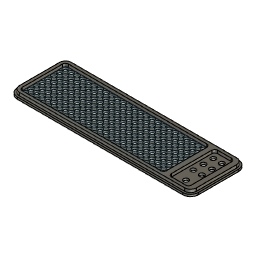
Frontal (Autodesk Fusion 360 design; units mm, degrees)
Autodesk Fusion 360 part; units mm, degrees
sketch "Boceto1" plane through (0, 0, 0) normal (0, 0, 1) x (1, 0, 0)
  circle A0 centre (2.9, 2.9) radius 2.5
  circle A1 centre (8.7, 2.9) radius 2.5
  circle A2 centre (20.3, 2.9) radius 2.5
  circle A3 centre (14.5, 2.9) radius 2.5
  circle A4 centre (43.5, 2.9) radius 2.5
  circle A5 centre (26.1, 2.9) radius 2.5
  circle A6 centre (31.9, 2.9) radius 2.5
  circle A7 centre (37.7, 2.9) radius 2.5
  circle A8 centre (55.1, 2.9) radius 2.5
  circle A9 centre (78.3, 2.9) radius 2.5
  circle A10 centre (84.1, 2.9) radius 2.5
  circle A11 centre (72.5, 2.9) radius 2.5
  circle A12 centre (89.9, 2.9) radius 2.5
  circle A13 centre (60.9, 2.9) radius 2.5
  circle A14 centre (66.7, 2.9) radius 2.5
  circle A15 centre (49.3, 2.9) radius 2.5
  circle A16 centre (118.9, 2.9) radius 2.5
  circle A17 centre (107.3, 2.9) radius 2.5
  circle A18 centre (95.7, 2.9) radius 2.5
  circle A19 centre (136.3, 2.9) radius 2.5
  circle A20 centre (113.1, 2.9) radius 2.5
  circle A21 centre (130.5, 2.9) radius 2.5
  circle A22 centre (124.7, 2.9) radius 2.5
  circle A23 centre (142.1, 2.9) radius 2.5
  circle A24 centre (101.5, 2.9) radius 2.5
  circle A25 centre (142.1, 8.7) radius 2.5
  circle A26 centre (66.7, 8.7) radius 2.5
  circle A27 centre (60.9, 8.7) radius 2.5
  circle A28 centre (2.9, 8.7) radius 2.5
  circle A29 centre (72.5, 8.7) radius 2.5
  circle A30 centre (130.5, 8.7) radius 2.5
  circle A31 centre (43.5, 8.7) radius 2.5
  circle A32 centre (20.3, 8.7) radius 2.5
  circle A33 centre (31.9, 8.7) radius 2.5
  circle A34 centre (101.5, 8.7) radius 2.5
  circle A35 centre (84.1, 8.7) radius 2.5
  circle A36 centre (113.1, 8.7) radius 2.5
  circle A37 centre (8.7, 8.7) radius 2.5
  circle A38 centre (55.1, 8.7) radius 2.5
  circle A39 centre (78.3, 8.7) radius 2.5
  circle A40 centre (124.7, 8.7) radius 2.5
  circle A41 centre (14.5, 8.7) radius 2.5
  circle A42 centre (26.1, 8.7) radius 2.5
  circle A43 centre (49.3, 8.7) radius 2.5
  circle A44 centre (89.9, 8.7) radius 2.5
  circle A45 centre (37.7, 8.7) radius 2.5
  circle A46 centre (136.3, 8.7) radius 2.5
  circle A47 centre (118.9, 8.7) radius 2.5
  circle A48 centre (107.3, 8.7) radius 2.5
  circle A49 centre (95.7, 8.7) radius 2.5
  circle A50 centre (78.3, 14.5) radius 2.5
  circle A51 centre (72.5, 14.5) radius 2.5
  circle A52 centre (26.1, 14.5) radius 2.5
  circle A53 centre (136.3, 20.3) radius 2.5
  circle A54 centre (37.7, 20.3) radius 2.5
  circle A55 centre (89.9, 20.3) radius 2.5
  circle A56 centre (49.3, 20.3) radius 2.5
  circle A57 centre (66.7, 14.5) radius 2.5
  circle A58 centre (113.1, 20.3) radius 2.5
  circle A59 centre (118.9, 20.3) radius 2.5
  circle A60 centre (124.7, 20.3) radius 2.5
  circle A61 centre (84.1, 20.3) radius 2.5
  circle A62 centre (20.3, 14.5) radius 2.5
  circle A63 centre (72.5, 20.3) radius 2.5
  circle A64 centre (142.1, 14.5) radius 2.5
  circle A65 centre (55.1, 14.5) radius 2.5
  circle A66 centre (14.5, 14.5) radius 2.5
  circle A67 centre (8.7, 20.3) radius 2.5
  circle A68 centre (101.5, 14.5) radius 2.5
  circle A69 centre (118.9, 14.5) radius 2.5
  circle A70 centre (2.9, 14.5) radius 2.5
  circle A71 centre (107.3, 14.5) radius 2.5
  circle A72 centre (8.7, 14.5) radius 2.5
  circle A73 centre (124.7, 14.5) radius 2.5
  circle A74 centre (113.1, 14.5) radius 2.5
  circle A75 centre (26.1, 20.3) radius 2.5
  circle A76 centre (49.3, 14.5) radius 2.5
  circle A77 centre (20.3, 20.3) radius 2.5
  circle A78 centre (66.7, 20.3) radius 2.5
  circle A79 centre (43.5, 14.5) radius 2.5
  circle A80 centre (43.5, 20.3) radius 2.5
  circle A81 centre (130.5, 20.3) radius 2.5
  circle A82 centre (78.3, 20.3) radius 2.5
  circle A83 centre (31.9, 14.5) radius 2.5
  circle A84 centre (89.9, 14.5) radius 2.5
  circle A85 centre (95.7, 20.3) radius 2.5
  circle A86 centre (55.1, 20.3) radius 2.5
  circle A87 centre (37.7, 14.5) radius 2.5
  circle A88 centre (31.9, 20.3) radius 2.5
  circle A89 centre (107.3, 20.3) radius 2.5
  circle A90 centre (101.5, 20.3) radius 2.5
  circle A91 centre (60.9, 20.3) radius 2.5
  circle A92 centre (130.5, 14.5) radius 2.5
  circle A93 centre (84.1, 14.5) radius 2.5
  circle A94 centre (14.5, 20.3) radius 2.5
  circle A95 centre (60.9, 14.5) radius 2.5
  circle A96 centre (2.9, 20.3) radius 2.5
  circle A97 centre (136.3, 14.5) radius 2.5
  circle A98 centre (142.1, 20.3) radius 2.5
  circle A99 centre (95.7, 14.5) radius 2.5
  circle A100 centre (55.1, 26.1) radius 2.5
  circle A101 centre (31.9, 31.9) radius 2.5
  circle A102 centre (95.7, 26.1) radius 2.5
  circle A103 centre (136.3, 26.1) radius 2.5
  circle A104 centre (43.5, 26.1) radius 2.5
  circle A105 centre (60.9, 26.1) radius 2.5
  circle A106 centre (8.7, 26.1) radius 2.5
  circle A107 centre (113.1, 31.9) radius 2.5
  circle A108 centre (49.3, 31.9) radius 2.5
  circle A109 centre (84.1, 26.1) radius 2.5
  circle A110 centre (49.3, 26.1) radius 2.5
  circle A111 centre (89.9, 26.1) radius 2.5
  circle A112 centre (130.5, 31.9) radius 2.5
  circle A113 centre (101.5, 31.9) radius 2.5
  circle A114 centre (31.9, 26.1) radius 2.5
  circle A115 centre (142.1, 31.9) radius 2.5
  circle A116 centre (8.7, 31.9) radius 2.5
  circle A117 centre (72.5, 26.1) radius 2.5
  circle A118 centre (78.3, 31.9) radius 2.5
  circle A119 centre (124.7, 31.9) radius 2.5
  circle A120 centre (118.9, 26.1) radius 2.5
  circle A121 centre (78.3, 26.1) radius 2.5
  circle A122 centre (66.7, 31.9) radius 2.5
  circle A123 centre (113.1, 26.1) radius 2.5
  circle A124 centre (142.1, 26.1) radius 2.5
  circle A125 centre (26.1, 31.9) radius 2.5
  circle A126 centre (60.9, 31.9) radius 2.5
  circle A127 centre (89.9, 31.9) radius 2.5
  circle A128 centre (26.1, 26.1) radius 2.5
  circle A129 centre (37.7, 26.1) radius 2.5
  circle A130 centre (72.5, 31.9) radius 2.5
  circle A131 centre (20.3, 26.1) radius 2.5
  circle A132 centre (14.5, 26.1) radius 2.5
  circle A133 centre (84.1, 31.9) radius 2.5
  circle A134 centre (136.3, 31.9) radius 2.5
  circle A135 centre (14.5, 31.9) radius 2.5
  circle A136 centre (124.7, 26.1) radius 2.5
  circle A137 centre (66.7, 26.1) radius 2.5
  circle A138 centre (101.5, 26.1) radius 2.5
  circle A139 centre (118.9, 31.9) radius 2.5
  circle A140 centre (43.5, 31.9) radius 2.5
  circle A141 centre (107.3, 31.9) radius 2.5
  circle A142 centre (55.1, 31.9) radius 2.5
  circle A143 centre (107.3, 26.1) radius 2.5
  circle A144 centre (20.3, 31.9) radius 2.5
  circle A145 centre (2.9, 31.9) radius 2.5
  circle A146 centre (2.9, 26.1) radius 2.5
  circle A147 centre (130.5, 26.1) radius 2.5
  circle A148 centre (95.7, 31.9) radius 2.5
  circle A149 centre (37.7, 31.9) radius 2.5
  circle A150 centre (84.1, 43.5) radius 2.5
  circle A151 centre (84.1, 37.7) radius 2.5
  circle A152 centre (72.5, 43.5) radius 2.5
  circle A153 centre (78.3, 37.7) radius 2.5
  circle A154 centre (89.9, 37.7) radius 2.5
  circle A155 centre (72.5, 37.7) radius 2.5
  circle A156 centre (78.3, 43.5) radius 2.5
  circle A157 centre (89.9, 43.5) radius 2.5
  circle A158 centre (95.7, 37.7) radius 2.5
  circle A159 centre (107.3, 37.7) radius 2.5
  circle A160 centre (107.3, 43.5) radius 2.5
  circle A161 centre (14.5, 37.7) radius 2.5
  circle A162 centre (43.5, 37.7) radius 2.5
  circle A163 centre (31.9, 43.5) radius 2.5
  circle A164 centre (66.7, 37.7) radius 2.5
  circle A165 centre (124.7, 43.5) radius 2.5
  circle A166 centre (101.5, 43.5) radius 2.5
  circle A167 centre (95.7, 43.5) radius 2.5
  circle A168 centre (8.7, 43.5) radius 2.5
  circle A169 centre (26.1, 37.7) radius 2.5
  circle A170 centre (113.1, 37.7) radius 2.5
  circle A171 centre (20.3, 43.5) radius 2.5
  circle A172 centre (113.1, 43.5) radius 2.5
  circle A173 centre (49.3, 37.7) radius 2.5
  circle A174 centre (37.7, 37.7) radius 2.5
  circle A175 centre (49.3, 43.5) radius 2.5
  circle A176 centre (2.9, 43.5) radius 2.5
  circle A177 centre (130.5, 43.5) radius 2.5
  circle A178 centre (118.9, 43.5) radius 2.5
  circle A179 centre (55.1, 43.5) radius 2.5
  circle A180 centre (66.7, 43.5) radius 2.5
  circle A181 centre (136.3, 43.5) radius 2.5
  circle A182 centre (60.9, 43.5) radius 2.5
  circle A183 centre (136.3, 37.7) radius 2.5
  circle A184 centre (142.1, 43.5) radius 2.5
  circle A185 centre (43.5, 43.5) radius 2.5
  circle A186 centre (101.5, 37.7) radius 2.5
  circle A187 centre (2.9, 37.7) radius 2.5
  circle A188 centre (20.3, 37.7) radius 2.5
  circle A189 centre (130.5, 37.7) radius 2.5
  circle A190 centre (14.5, 43.5) radius 2.5
  circle A191 centre (37.7, 43.5) radius 2.5
  circle A192 centre (118.9, 37.7) radius 2.5
  circle A193 centre (55.1, 37.7) radius 2.5
  circle A194 centre (31.9, 37.7) radius 2.5
  circle A195 centre (124.7, 37.7) radius 2.5
  circle A196 centre (60.9, 37.7) radius 2.5
  circle A197 centre (142.1, 37.7) radius 2.5
  circle A198 centre (26.1, 43.5) radius 2.5
  circle A199 centre (8.7, 37.7) radius 2.5
  line L0 (2.9, 0) -> (142.1, 0)
  line L1 (145, 2.9) -> (145, 43.5)
  line L2 (0, 43.5) -> (0, 2.9)
  line L3 (-2.9, 43.5) -> (-2.9, 2.9)
  line L4 (2.9, -2.9) -> (169.2, -2.9)
  line L5 (142.1, 46.4) -> (2.9, 46.4)
  line L6 (175, 2.9) -> (175, 43.5)
  line L7 (169.2, 49.3) -> (2.9, 49.3)
  arc A200 (2.9, 49.3) -> (-2.9, 43.5) centre (2.9, 43.5) ccw
  arc A201 (-2.9, 2.9) -> (2.9, -2.9) centre (2.9, 2.9) ccw
  arc A202 (169.2, -2.9) -> (175, 2.9) centre (169.2, 2.9) ccw
  arc A203 (175, 43.5) -> (169.2, 49.3) centre (169.2, 43.5) ccw
  arc A204 (2.9, 46.4) -> (0, 43.5) centre (2.9, 43.5) ccw
  arc A205 (0, 2.9) -> (2.9, 0) centre (2.9, 2.9) ccw
  arc A206 (142.1, 0) -> (145, 2.9) centre (142.1, 2.9) ccw
  arc A207 (145, 43.5) -> (142.1, 46.4) centre (142.1, 43.5) ccw
  line L8 (170, 2.4388) -> (170, 43.0388)
  line L9 (166.6388, 46.4) -> (152.9, 46.4)
  arc A208 (170, 43.0388) -> (166.6388, 46.4) centre (166.6388, 43.0388) ccw
  arc A209 (167.5612, 0) -> (170, 2.4388) centre (167.5612, 2.4388) ccw
  line L10 (152.9, 0) -> (167.5612, 0)
  line L11 (150, 43.5) -> (150, 2.9)
  arc A210 (152.9, 46.4) -> (150, 43.5) centre (152.9, 43.5) ccw
  arc A211 (150, 2.9) -> (152.9, 0) centre (152.9, 2.9) ccw
  circle A212 centre (155, 20) radius 2.5
  circle A213 centre (155, 30) radius 2.5
  circle A214 centre (155, 40) radius 2.5
  circle A215 centre (160, 7.5) radius 2.5
  circle A216 centre (155, 20) radius 2.5
  circle A217 centre (155, 30) radius 2.5
  circle A218 centre (155, 40) radius 2.5
  circle A219 centre (163.5, 20) radius 2.5
  circle A220 centre (163.5, 30) radius 2.5
  circle A221 centre (163.5, 40) radius 2.5
  circle A222 centre (101.5, 120.3) radius 2.5
  circle A223 centre (89.9, 126.1) radius 2.5
  line L12 (2.9, 97.1) -> (169.2, 97.1)
  circle A224 centre (89.9, 114.5) radius 2.5
  line L13 (142.1, 146.4) -> (2.9, 146.4)
  circle A225 centre (95.7, 120.3) radius 2.5
  circle A226 centre (95.7, 143.5) radius 2.5
  circle A227 centre (89.9, 143.5) radius 2.5
  circle A228 centre (101.5, 114.5) radius 2.5
  circle A229 centre (55.1, 137.7) radius 2.5
  circle A230 centre (107.3, 102.9) radius 2.5
  circle A231 centre (43.5, 126.1) radius 2.5
  circle A232 centre (55.1, 131.9) radius 2.5
  circle A233 centre (101.5, 108.7) radius 2.5
  circle A234 centre (89.9, 137.7) radius 2.5
  circle A235 centre (101.5, 102.9) radius 2.5
  circle A236 centre (107.3, 108.7) radius 2.5
  circle A237 centre (124.7, 114.5) radius 2.5
  circle A238 centre (2.9, 126.1) radius 2.5
  circle A239 centre (124.7, 131.9) radius 2.5
  circle A240 centre (60.9, 102.9) radius 2.5
  circle A241 centre (84.1, 126.1) radius 2.5
  circle A242 centre (78.3, 114.5) radius 2.5
  circle A243 centre (155, 130) radius 2.5
  circle A244 centre (136.3, 143.5) radius 2.5
  circle A245 centre (118.9, 114.5) radius 2.5
  circle A246 centre (14.5, 131.9) radius 2.5
  circle A247 centre (113.1, 143.5) radius 2.5
  circle A248 centre (155, 140) radius 2.5
  circle A249 centre (163.5, 130) radius 2.5
  circle A250 centre (130.5, 120.3) radius 2.5
  circle A251 centre (142.1, 143.5) radius 2.5
  circle A252 centre (136.3, 114.5) radius 2.5
  circle A253 centre (26.1, 126.1) radius 2.5
  circle A254 centre (130.5, 126.1) radius 2.5
  arc A255 (-2.9, 102.9) -> (2.9, 97.1) centre (2.9, 102.9) ccw
  circle A256 centre (101.5, 126.1) radius 2.5
  circle A257 centre (142.1, 102.9) radius 2.5
  circle A258 centre (142.1, 131.9) radius 2.5
  circle A259 centre (160, 107.5) radius 2.5
  circle A260 centre (78.3, 102.9) radius 2.5
  circle A261 centre (49.3, 120.3) radius 2.5
  circle A262 centre (118.9, 137.7) radius 2.5
  circle A263 centre (20.3, 137.7) radius 2.5
  circle A264 centre (142.1, 120.3) radius 2.5
  circle A265 centre (26.1, 131.9) radius 2.5
  circle A266 centre (118.9, 126.1) radius 2.5
  circle A267 centre (142.1, 137.7) radius 2.5
  line L14 (170, 102.4388) -> (170, 143.0388)
  circle A268 centre (124.7, 143.5) radius 2.5
  arc A269 (2.9, 149.3) -> (-2.9, 143.5) centre (2.9, 143.5) ccw
  circle A270 centre (118.9, 120.3) radius 2.5
  circle A271 centre (130.5, 108.7) radius 2.5
  circle A272 centre (8.7, 108.7) radius 2.5
  circle A273 centre (118.9, 131.9) radius 2.5
  circle A274 centre (8.7, 126.1) radius 2.5
  circle A275 centre (66.7, 114.5) radius 2.5
  circle A276 centre (84.1, 108.7) radius 2.5
  circle A277 centre (8.7, 131.9) radius 2.5
  circle A278 centre (113.1, 131.9) radius 2.5
  arc A279 (142.1, 100) -> (145, 102.9) centre (142.1, 102.9) ccw
  circle A280 centre (31.9, 120.3) radius 2.5
  circle A281 centre (142.1, 108.7) radius 2.5
  line L15 (-2.9, 143.5) -> (-2.9, 102.9)
  circle A282 centre (2.9, 137.7) radius 2.5
  circle A283 centre (136.3, 102.9) radius 2.5
  circle A284 centre (8.7, 120.3) radius 2.5
  circle A285 centre (20.3, 108.7) radius 2.5
  circle A286 centre (31.9, 131.9) radius 2.5
  circle A287 centre (136.3, 120.3) radius 2.5
  circle A288 centre (130.5, 131.9) radius 2.5
  circle A289 centre (155, 120) radius 2.5
  circle A290 centre (14.5, 137.7) radius 2.5
  circle A291 centre (130.5, 114.5) radius 2.5
  circle A292 centre (26.1, 102.9) radius 2.5
  circle A293 centre (14.5, 108.7) radius 2.5
  circle A294 centre (14.5, 102.9) radius 2.5
  circle A295 centre (20.3, 102.9) radius 2.5
  circle A296 centre (2.9, 108.7) radius 2.5
  arc A297 (167.5612, 100) -> (170, 102.4388) centre (167.5612, 102.4388) ccw
  circle A298 centre (124.7, 102.9) radius 2.5
  arc A299 (150, 102.9) -> (152.9, 100) centre (152.9, 102.9) ccw
  circle A300 centre (26.1, 120.3) radius 2.5
  circle A301 centre (31.9, 108.7) radius 2.5
  circle A302 centre (26.1, 114.5) radius 2.5
  circle A303 centre (113.1, 108.7) radius 2.5
  arc A304 (169.2, 97.1) -> (175, 102.9) centre (169.2, 102.9) ccw
  line L16 (152.9, 100) -> (167.5612, 100)
  circle A305 centre (118.9, 108.7) radius 2.5
  circle A306 centre (20.3, 120.3) radius 2.5
  circle A307 centre (8.7, 102.9) radius 2.5
  circle A308 centre (163.5, 120) radius 2.5
  circle A309 centre (8.7, 114.5) radius 2.5
  arc A310 (175, 143.5) -> (169.2, 149.3) centre (169.2, 143.5) ccw
  circle A311 centre (118.9, 102.9) radius 2.5
  circle A312 centre (113.1, 120.3) radius 2.5
  circle A313 centre (124.7, 120.3) radius 2.5
  arc A314 (0, 102.9) -> (2.9, 100) centre (2.9, 102.9) ccw
  circle A315 centre (20.3, 114.5) radius 2.5
  circle A316 centre (155, 120) radius 2.5
  circle A317 centre (136.3, 137.7) radius 2.5
  circle A318 centre (124.7, 126.1) radius 2.5
  circle A319 centre (14.5, 120.3) radius 2.5
  circle A320 centre (163.5, 140) radius 2.5
  circle A321 centre (136.3, 131.9) radius 2.5
  circle A322 centre (14.5, 114.5) radius 2.5
  circle A323 centre (130.5, 102.9) radius 2.5
  circle A324 centre (136.3, 108.7) radius 2.5
  circle A325 centre (124.7, 137.7) radius 2.5
  circle A326 centre (124.7, 108.7) radius 2.5
  circle A327 centre (142.1, 114.5) radius 2.5
  circle A328 centre (26.1, 108.7) radius 2.5
  circle A329 centre (118.9, 143.5) radius 2.5
  circle A330 centre (155, 140) radius 2.5
  circle A331 centre (31.9, 114.5) radius 2.5
  circle A332 centre (2.9, 114.5) radius 2.5
  circle A333 centre (2.9, 120.3) radius 2.5
  circle A334 centre (113.1, 114.5) radius 2.5
  arc A335 (170, 143.0388) -> (166.6388, 146.4) centre (166.6388, 143.0388) ccw
  circle A336 centre (95.7, 137.7) radius 2.5
  circle A337 centre (66.7, 108.7) radius 2.5
  circle A338 centre (130.5, 143.5) radius 2.5
  circle A339 centre (43.5, 143.5) radius 2.5
  circle A340 centre (78.3, 120.3) radius 2.5
  circle A341 centre (37.7, 114.5) radius 2.5
  line L17 (175, 102.9) -> (175, 143.5)
  circle A342 centre (37.7, 137.7) radius 2.5
  circle A343 centre (66.7, 143.5) radius 2.5
  circle A344 centre (60.9, 126.1) radius 2.5
  circle A345 centre (55.1, 126.1) radius 2.5
  circle A346 centre (20.3, 131.9) radius 2.5
  circle A347 centre (84.1, 143.5) radius 2.5
  circle A348 centre (101.5, 143.5) radius 2.5
  circle A349 centre (95.7, 114.5) radius 2.5
  circle A350 centre (2.9, 143.5) radius 2.5
  circle A351 centre (49.3, 102.9) radius 2.5
  arc A352 (145, 143.5) -> (142.1, 146.4) centre (142.1, 143.5) ccw
  circle A353 centre (14.5, 143.5) radius 2.5
  circle A354 centre (84.1, 102.9) radius 2.5
  circle A355 centre (60.9, 143.5) radius 2.5
  circle A356 centre (107.3, 143.5) radius 2.5
  circle A357 centre (60.9, 120.3) radius 2.5
  circle A358 centre (49.3, 131.9) radius 2.5
  circle A359 centre (55.1, 108.7) radius 2.5
  circle A360 centre (2.9, 131.9) radius 2.5
  circle A361 centre (142.1, 126.1) radius 2.5
  circle A362 centre (43.5, 108.7) radius 2.5
  circle A363 centre (60.9, 137.7) radius 2.5
  circle A364 centre (107.3, 137.7) radius 2.5
  circle A365 centre (8.7, 137.7) radius 2.5
  circle A366 centre (49.3, 143.5) radius 2.5
  circle A367 centre (60.9, 131.9) radius 2.5
  circle A368 centre (72.5, 137.7) radius 2.5
  circle A369 centre (72.5, 114.5) radius 2.5
  circle A370 centre (55.1, 102.9) radius 2.5
  circle A371 centre (89.9, 131.9) radius 2.5
  circle A372 centre (72.5, 131.9) radius 2.5
  circle A373 centre (72.5, 120.3) radius 2.5
  circle A374 centre (66.7, 120.3) radius 2.5
  circle A375 centre (95.7, 131.9) radius 2.5
  line L18 (166.6388, 146.4) -> (152.9, 146.4)
  circle A376 centre (66.7, 102.9) radius 2.5
  circle A377 centre (26.1, 143.5) radius 2.5
  line L19 (0, 143.5) -> (0, 102.9)
  circle A378 centre (84.1, 120.3) radius 2.5
  circle A379 centre (43.5, 114.5) radius 2.5
  arc A380 (152.9, 146.4) -> (150, 143.5) centre (152.9, 143.5) ccw
  circle A381 centre (20.3, 126.1) radius 2.5
  line L20 (150, 143.5) -> (150, 102.9)
  line L21 (145, 102.9) -> (145, 143.5)
  circle A382 centre (37.7, 102.9) radius 2.5
  circle A383 centre (37.7, 120.3) radius 2.5
  circle A384 centre (26.1, 137.7) radius 2.5
  circle A385 centre (31.9, 126.1) radius 2.5
  circle A386 centre (66.7, 137.7) radius 2.5
  circle A387 centre (37.7, 143.5) radius 2.5
  circle A388 centre (31.9, 143.5) radius 2.5
  circle A389 centre (101.5, 137.7) radius 2.5
  circle A390 centre (55.1, 143.5) radius 2.5
  circle A391 centre (113.1, 137.7) radius 2.5
  circle A392 centre (84.1, 114.5) radius 2.5
  circle A393 centre (43.5, 120.3) radius 2.5
  circle A394 centre (72.5, 102.9) radius 2.5
  circle A395 centre (155, 130) radius 2.5
  circle A396 centre (78.3, 126.1) radius 2.5
  circle A397 centre (37.7, 108.7) radius 2.5
  circle A398 centre (66.7, 131.9) radius 2.5
  circle A399 centre (49.3, 108.7) radius 2.5
  circle A400 centre (43.5, 131.9) radius 2.5
  circle A401 centre (72.5, 126.1) radius 2.5
  circle A402 centre (101.5, 131.9) radius 2.5
  circle A403 centre (49.3, 126.1) radius 2.5
  arc A404 (2.9, 146.4) -> (0, 143.5) centre (2.9, 143.5) ccw
  circle A405 centre (113.1, 126.1) radius 2.5
  circle A406 centre (78.3, 131.9) radius 2.5
  circle A407 centre (78.3, 143.5) radius 2.5
  circle A408 centre (43.5, 102.9) radius 2.5
  circle A409 centre (72.5, 143.5) radius 2.5
  circle A410 centre (84.1, 131.9) radius 2.5
  circle A411 centre (43.5, 137.7) radius 2.5
  circle A412 centre (78.3, 137.7) radius 2.5
  circle A413 centre (31.9, 137.7) radius 2.5
  circle A414 centre (49.3, 137.7) radius 2.5
  circle A415 centre (20.3, 143.5) radius 2.5
  circle A416 centre (55.1, 114.5) radius 2.5
  circle A417 centre (89.9, 108.7) radius 2.5
  circle A418 centre (107.3, 120.3) radius 2.5
  circle A419 centre (72.5, 108.7) radius 2.5
  circle A420 centre (49.3, 114.5) radius 2.5
  circle A421 centre (130.5, 137.7) radius 2.5
  circle A422 centre (8.7, 143.5) radius 2.5
  circle A423 centre (136.3, 126.1) radius 2.5
  circle A424 centre (60.9, 108.7) radius 2.5
  circle A425 centre (78.3, 108.7) radius 2.5
  circle A426 centre (95.7, 126.1) radius 2.5
  circle A427 centre (107.3, 131.9) radius 2.5
  circle A428 centre (60.9, 114.5) radius 2.5
  circle A429 centre (37.7, 126.1) radius 2.5
  circle A430 centre (66.7, 126.1) radius 2.5
  circle A431 centre (14.5, 126.1) radius 2.5
  circle A432 centre (107.3, 126.1) radius 2.5
  circle A433 centre (37.7, 131.9) radius 2.5
  circle A434 centre (55.1, 120.3) radius 2.5
  circle A435 centre (84.1, 137.7) radius 2.5
  circle A436 centre (2.9, 102.9) radius 2.5
  circle A437 centre (31.9, 102.9) radius 2.5
  circle A438 centre (113.1, 102.9) radius 2.5
  circle A439 centre (89.9, 120.3) radius 2.5
  line L22 (169.2, 149.3) -> (2.9, 149.3)
  line L23 (2.9, 100) -> (142.1, 100)
  circle A440 centre (95.7, 108.7) radius 2.5
  circle A441 centre (89.9, 102.9) radius 2.5
  circle A442 centre (95.7, 102.9) radius 2.5
  circle A443 centre (107.3, 114.5) radius 2.5
  point P0 (0, 100)
  constraint horizontal L0
  constraint vertical L1
  constraint vertical L2
  constraint vertical L3
  constraint horizontal L4
  constraint horizontal L5
  constraint vertical L6
  constraint horizontal L7
  constraint tangent L3 A200
  constraint tangent L7 A200
  constraint tangent L4 A201
  constraint tangent L3 A201
  constraint tangent L4 A202
  constraint tangent L6 A202
  constraint tangent L7 A203
  constraint tangent L6 A203
  constraint tangent L2 A204
  constraint tangent L5 A204
  constraint tangent L2 A205
  constraint tangent L0 A205
  constraint tangent L0 A206
  constraint tangent L1 A206
  constraint tangent L5 A207
  constraint tangent L1 A207
  constraint horizontal L10
  constraint vertical L8
  constraint horizontal L9
  constraint tangent A209 L10
  constraint tangent L8 A209
  constraint tangent L9 A208
  constraint tangent L8 A208
  constraint vertical L11
  constraint tangent L11 A210
  constraint tangent L11 A211
  constraint coincident L0 L10.start
  constraint horizontal L23
  constraint vertical L21
  constraint vertical L19
  constraint vertical L15
  constraint horizontal L12
  constraint horizontal L13
  constraint vertical L17
  constraint horizontal L22
  constraint tangent A269 L15
  constraint tangent A269 L22
  constraint tangent L12 A255
  constraint tangent A255 L15
  constraint tangent L12 A304
  constraint tangent A304 L17
  constraint tangent A310 L22
  constraint tangent A310 L17
  constraint tangent L19 A404
  constraint tangent L13 A404
  constraint tangent A314 L19
  constraint tangent A314 L23
  constraint tangent A279 L23
  constraint tangent A279 L21
  constraint tangent L13 A352
  constraint tangent A352 L21
  constraint horizontal L16
  constraint vertical L14
  constraint horizontal L18
  constraint tangent A297 L16
  constraint tangent L14 A297
  constraint tangent A335 L18
  constraint tangent L14 A335
  constraint vertical L20
  constraint tangent A380 L20
  constraint tangent A299 L20
  constraint coincident A299.end L23
extrude "Extruir1" add sketch "Boceto1" along normal blind 2 contours L3 L4 L6 L7 A200 A201 A202 A203 | L13 A279 A314 A352 L19 L21 A404 L23 | L14 A297 A299 L16 A335 L18 A380 L20 makes body 1 at (173.3333, 29.8129, 0) makes body 2 at (133.0442, 111.9999, 0) makes body 3 at (153.787, 109.6573, 0)
extrude "Extruir2" add 1 faces at (173.3333, 29.8129, 2) along direction (0, 0, 1) blind 3 on bodies 1 bodies 1
move_body "Desplazar1" bodies 2 3 to x (1, 0, 0) y (0, 1, 0) z (0, 0, 1) at (0, -100, 0)
combine "Combinar1" operation add target body 2 tool bodies 1 3
sketch "Boceto2" plane through (0, 0, 2) normal (0, 0, 1) x (-1, 0, 0)
  circle A0 centre (-101.5, -8.7) radius 2.5
  circle A1 centre (-2.9, -14.5) radius 2.5
  circle A2 centre (-37.7, -8.7) radius 2.5
  circle A3 centre (-142.1, -26.1) radius 2.5
  circle A4 centre (-136.3, -26.1) radius 2.5
  circle A5 centre (-78.3, -20.3) radius 2.5
  circle A6 centre (-60.9, -2.9) radius 2.5
  circle A7 centre (-43.5, -43.5) radius 2.5
  circle A8 centre (-130.5, -43.5) radius 2.5
  circle A9 centre (-43.5, -2.9) radius 2.5
  circle A10 centre (-43.5, -31.9) radius 2.5
  circle A11 centre (-107.3, -31.9) radius 2.5
  circle A12 centre (-66.7, -8.7) radius 2.5
  circle A13 centre (-95.7, -37.7) radius 2.5
  circle A14 centre (-118.9, -37.7) radius 2.5
  circle A15 centre (-49.3, -20.3) radius 2.5
  circle A16 centre (-20.3, -26.1) radius 2.5
  circle A17 centre (-66.7, -37.7) radius 2.5
  circle A18 centre (-124.7, -14.5) radius 2.5
  circle A19 centre (-113.1, -14.5) radius 2.5
  circle A20 centre (-2.9, -20.3) radius 2.5
  circle A21 centre (-31.9, -14.5) radius 2.5
  circle A22 centre (-31.9, -43.5) radius 2.5
  circle A23 centre (-72.5, -43.5) radius 2.5
  circle A24 centre (-118.9, -26.1) radius 2.5
  circle A25 centre (-95.7, -26.1) radius 2.5
  circle A26 centre (-118.9, -43.5) radius 2.5
  circle A27 centre (-26.1, -8.7) radius 2.5
  circle A28 centre (-55.1, -31.9) radius 2.5
  circle A29 centre (-107.3, -20.3) radius 2.5
  circle A30 centre (-142.1, -14.5) radius 2.5
  circle A31 centre (-118.9, -14.5) radius 2.5
  circle A32 centre (-124.7, -8.7) radius 2.5
  circle A33 centre (-72.5, -20.3) radius 2.5
  circle A34 centre (-124.7, -37.7) radius 2.5
  circle A35 centre (-84.1, -31.9) radius 2.5
  circle A36 centre (-136.3, -8.7) radius 2.5
  circle A37 centre (-130.5, -2.9) radius 2.5
  circle A38 centre (-101.5, -20.3) radius 2.5
  circle A39 centre (-14.5, -14.5) radius 2.5
  circle A40 centre (-60.9, -8.7) radius 2.5
  circle A41 centre (-43.5, -8.7) radius 2.5
  circle A42 centre (-136.3, -31.9) radius 2.5
  circle A43 centre (-72.5, -8.7) radius 2.5
  circle A44 centre (-107.3, -8.7) radius 2.5
  circle A45 centre (-124.7, -43.5) radius 2.5
  circle A46 centre (-72.5, -31.9) radius 2.5
  circle A47 centre (-14.5, -20.3) radius 2.5
  circle A48 centre (-66.7, -20.3) radius 2.5
  circle A49 centre (-124.7, -26.1) radius 2.5
  circle A50 centre (-72.5, -2.9) radius 2.5
  circle A51 centre (-26.1, -31.9) radius 2.5
  circle A52 centre (-136.3, -37.7) radius 2.5
  circle A53 centre (-37.7, -20.3) radius 2.5
  circle A54 centre (-101.5, -37.7) radius 2.5
  circle A55 centre (-20.3, -14.5) radius 2.5
  circle A56 centre (-60.9, -20.3) radius 2.5
  circle A57 centre (-142.1, -2.9) radius 2.5
  circle A58 centre (-124.7, -20.3) radius 2.5
  circle A59 centre (-89.9, -26.1) radius 2.5
  circle A60 centre (-8.7, -43.5) radius 2.5
  circle A61 centre (-60.9, -37.7) radius 2.5
  circle A62 centre (-113.1, -20.3) radius 2.5
  circle A63 centre (-130.5, -37.7) radius 2.5
  circle A64 centre (-89.9, -31.9) radius 2.5
  circle A65 centre (-118.9, -2.9) radius 2.5
  circle A66 centre (-84.1, -26.1) radius 2.5
  circle A67 centre (-118.9, -31.9) radius 2.5
  circle A68 centre (-95.7, -31.9) radius 2.5
  circle A69 centre (-8.7, -14.5) radius 2.5
  circle A70 centre (-113.1, -43.5) radius 2.5
  circle A71 centre (-43.5, -20.3) radius 2.5
  circle A72 centre (-113.1, -37.7) radius 2.5
  circle A73 centre (-8.7, -2.9) radius 2.5
  circle A74 centre (-101.5, -2.9) radius 2.5
  circle A75 centre (-20.3, -20.3) radius 2.5
  circle A76 centre (-130.5, -8.7) radius 2.5
  circle A77 centre (-118.9, -8.7) radius 2.5
  circle A78 centre (-8.7, -37.7) radius 2.5
  circle A79 centre (-101.5, -26.1) radius 2.5
  circle A80 centre (-49.3, -31.9) radius 2.5
  circle A81 centre (-113.1, -8.7) radius 2.5
  circle A82 centre (-55.1, -14.5) radius 2.5
  circle A83 centre (-95.7, -20.3) radius 2.5
  circle A84 centre (-26.1, -14.5) radius 2.5
  circle A85 centre (-31.9, -8.7) radius 2.5
  circle A86 centre (-55.1, -2.9) radius 2.5
  circle A87 centre (-55.1, -37.7) radius 2.5
  circle A88 centre (-84.1, -20.3) radius 2.5
  circle A89 centre (-26.1, -20.3) radius 2.5
  circle A90 centre (-43.5, -26.1) radius 2.5
  circle A91 centre (-124.7, -2.9) radius 2.5
  circle A92 centre (-2.9, -8.7) radius 2.5
  circle A93 centre (-136.3, -43.5) radius 2.5
  circle A94 centre (-31.9, -37.7) radius 2.5
  circle A95 centre (-43.5, -37.7) radius 2.5
  circle A96 centre (-20.3, -2.9) radius 2.5
  circle A97 centre (-2.9, -26.1) radius 2.5
  circle A98 centre (-43.5, -14.5) radius 2.5
  circle A99 centre (-95.7, -43.5) radius 2.5
  circle A100 centre (-14.5, -2.9) radius 2.5
  circle A101 centre (-55.1, -8.7) radius 2.5
  circle A102 centre (-14.5, -8.7) radius 2.5
  circle A103 centre (-26.1, -37.7) radius 2.5
  circle A104 centre (-26.1, -2.9) radius 2.5
  circle A105 centre (-130.5, -14.5) radius 2.5
  circle A106 centre (-66.7, -14.5) radius 2.5
  circle A107 centre (-49.3, -14.5) radius 2.5
  circle A108 centre (-14.5, -26.1) radius 2.5
  circle A109 centre (-14.5, -37.7) radius 2.5
  circle A110 centre (-8.7, -8.7) radius 2.5
  circle A111 centre (-89.9, -37.7) radius 2.5
  circle A112 centre (-72.5, -14.5) radius 2.5
  circle A113 centre (-130.5, -31.9) radius 2.5
  circle A114 centre (-14.5, -31.9) radius 2.5
  circle A115 centre (-136.3, -20.3) radius 2.5
  circle A116 centre (-49.3, -8.7) radius 2.5
  circle A117 centre (-101.5, -14.5) radius 2.5
  circle A118 centre (-14.5, -43.5) radius 2.5
  circle A119 centre (-84.1, -14.5) radius 2.5
  circle A120 centre (-101.5, -31.9) radius 2.5
  circle A121 centre (-84.1, -2.9) radius 2.5
  circle A122 centre (-49.3, -37.7) radius 2.5
  circle A123 centre (-37.7, -26.1) radius 2.5
  circle A124 centre (-95.7, -2.9) radius 2.5
  circle A125 centre (-95.7, -8.7) radius 2.5
  circle A126 centre (-89.9, -20.3) radius 2.5
  circle A127 centre (-113.1, -2.9) radius 2.5
  circle A128 centre (-107.3, -26.1) radius 2.5
  circle A129 centre (-2.9, -2.9) radius 2.5
  circle A130 centre (-89.9, -2.9) radius 2.5
  circle A131 centre (-84.1, -37.7) radius 2.5
  circle A132 centre (-37.7, -31.9) radius 2.5
  circle A133 centre (-55.1, -20.3) radius 2.5
  circle A134 centre (-31.9, -2.9) radius 2.5
  circle A135 centre (-107.3, -14.5) radius 2.5
  circle A136 centre (-101.5, -43.5) radius 2.5
  circle A137 centre (-20.3, -37.7) radius 2.5
  circle A138 centre (-107.3, -43.5) radius 2.5
  circle A139 centre (-26.1, -26.1) radius 2.5
  circle A140 centre (-8.7, -31.9) radius 2.5
  circle A141 centre (-107.3, -2.9) radius 2.5
  circle A142 centre (-84.1, -8.7) radius 2.5
  circle A143 centre (-142.1, -8.7) radius 2.5
  circle A144 centre (-55.1, -43.5) radius 2.5
  circle A145 centre (-113.1, -26.1) radius 2.5
  circle A146 centre (-78.3, -37.7) radius 2.5
  circle A147 centre (-66.7, -31.9) radius 2.5
  circle A148 centre (-136.3, -2.9) radius 2.5
  circle A149 centre (-72.5, -37.7) radius 2.5
  circle A150 centre (-84.1, -43.5) radius 2.5
  circle A151 centre (-49.3, -2.9) radius 2.5
  circle A152 centre (-113.1, -31.9) radius 2.5
  circle A153 centre (-78.3, -31.9) radius 2.5
  circle A154 centre (-78.3, -43.5) radius 2.5
  circle A155 centre (-66.7, -26.1) radius 2.5
  circle A156 centre (-49.3, -43.5) radius 2.5
  circle A157 centre (-31.9, -26.1) radius 2.5
  circle A158 centre (-2.9, -31.9) radius 2.5
  circle A159 centre (-31.9, -31.9) radius 2.5
  circle A160 centre (-37.7, -2.9) radius 2.5
  circle A161 centre (-89.9, -14.5) radius 2.5
  circle A162 centre (-95.7, -14.5) radius 2.5
  circle A163 centre (-78.3, -8.7) radius 2.5
  circle A164 centre (-66.7, -2.9) radius 2.5
  circle A165 centre (-130.5, -20.3) radius 2.5
  circle A166 centre (-37.7, -37.7) radius 2.5
  circle A167 centre (-60.9, -43.5) radius 2.5
  circle A168 centre (-78.3, -2.9) radius 2.5
  circle A169 centre (-89.9, -8.7) radius 2.5
  circle A170 centre (-20.3, -31.9) radius 2.5
  circle A171 centre (-60.9, -31.9) radius 2.5
  circle A172 centre (-31.9, -20.3) radius 2.5
  circle A173 centre (-60.9, -26.1) radius 2.5
  circle A174 centre (-49.3, -26.1) radius 2.5
  circle A175 centre (-124.7, -31.9) radius 2.5
  circle A176 centre (-107.3, -37.7) radius 2.5
  circle A177 centre (-130.5, -26.1) radius 2.5
  circle A178 centre (-37.7, -14.5) radius 2.5
  circle A179 centre (-142.1, -37.7) radius 2.5
  circle A180 centre (-78.3, -14.5) radius 2.5
  circle A181 centre (-8.7, -20.3) radius 2.5
  circle A182 centre (-142.1, -43.5) radius 2.5
  circle A183 centre (-78.3, -26.1) radius 2.5
  circle A184 centre (-136.3, -14.5) radius 2.5
  circle A185 centre (-8.7, -26.1) radius 2.5
  circle A186 centre (-26.1, -43.5) radius 2.5
  circle A187 centre (-55.1, -26.1) radius 2.5
  circle A188 centre (-60.9, -14.5) radius 2.5
  circle A189 centre (-66.7, -43.5) radius 2.5
  circle A190 centre (-142.1, -31.9) radius 2.5
  circle A191 centre (-72.5, -26.1) radius 2.5
  circle A192 centre (-37.7, -43.5) radius 2.5
  circle A193 centre (-2.9, -37.7) radius 2.5
  circle A194 centre (-20.3, -8.7) radius 2.5
  circle A195 centre (-2.9, -43.5) radius 2.5
  circle A196 centre (-20.3, -43.5) radius 2.5
  circle A197 centre (-89.9, -43.5) radius 2.5
  circle A198 centre (-142.1, -20.3) radius 2.5
  circle A199 centre (-118.9, -20.3) radius 2.5
  line L0 (-2.9, 0) -> (-142.1, 0)
  arc A200 (-142.1, 0) -> (-145, -2.9) centre (-142.1, -2.9) ccw
  line L1 (-145, -2.9) -> (-145, -43.5)
  arc A201 (-145, -43.5) -> (-142.1, -46.4) centre (-142.1, -43.5) ccw
  line L2 (-142.1, -46.4) -> (-2.9, -46.4)
  arc A202 (-2.9, -46.4) -> (0, -43.5) centre (-2.9, -43.5) ccw
  line L3 (0, -43.5) -> (0, -2.9)
  arc A203 (0, -2.9) -> (-2.9, 0) centre (-2.9, -2.9) ccw
sketch "Boceto3" plane through (0, 0, 0) normal (0, 0, 1) x (1, 0, 0)
sketch "Boceto4" plane through (0, 0, 0) normal (0, 0, 1) x (1, 0, 0)
  circle A0 centre (26.1, 14.5) radius 2.5
  circle A1 centre (8.7, 20.3) radius 2.5
  line L0 (152.9, 0) -> (167.5612, 0)
  circle A2 centre (155, 20) radius 2.5
  circle A3 centre (130.5, 20.3) radius 2.5
  circle A4 centre (2.9, 2.9) radius 2.5
  circle A5 centre (160, 7.5) radius 2.5
  circle A6 centre (130.5, 2.9) radius 2.5
  circle A7 centre (14.5, 2.9) radius 2.5
  circle A8 centre (37.7, 20.3) radius 2.5
  circle A9 centre (136.3, 20.3) radius 2.5
  arc A10 (142.1, 0) -> (145, 2.9) centre (142.1, 2.9) ccw
  arc A11 (0, 2.9) -> (2.9, 0) centre (2.9, 2.9) ccw
  circle A12 centre (8.7, 14.5) radius 2.5
  circle A13 centre (20.3, 20.3) radius 2.5
  circle A14 centre (8.7, 8.7) radius 2.5
  circle A15 centre (8.7, 2.9) radius 2.5
  circle A16 centre (78.3, 2.9) radius 2.5
  circle A17 centre (84.1, 8.7) radius 2.5
  circle A18 centre (130.5, 8.7) radius 2.5
  circle A19 centre (95.7, 20.3) radius 2.5
  circle A20 centre (37.7, 14.5) radius 2.5
  circle A21 centre (142.1, 2.9) radius 2.5
  circle A22 centre (31.9, 14.5) radius 2.5
  circle A23 centre (142.1, 8.7) radius 2.5
  circle A24 centre (95.7, 2.9) radius 2.5
  circle A25 centre (20.3, 14.5) radius 2.5
  circle A26 centre (60.9, 14.5) radius 2.5
  circle A27 centre (89.9, 2.9) radius 2.5
  circle A28 centre (2.9, 20.3) radius 2.5
  arc A29 (-2.9, 2.9) -> (2.9, -2.9) centre (2.9, 2.9) ccw
  circle A30 centre (95.7, 43.5) radius 2.5
  circle A31 centre (31.9, 31.9) radius 2.5
  circle A32 centre (124.7, 31.9) radius 2.5
  circle A33 centre (142.1, 20.3) radius 2.5
  circle A34 centre (26.1, 20.3) radius 2.5
  circle A35 centre (89.9, 14.5) radius 2.5
  circle A36 centre (124.7, 20.3) radius 2.5
  circle A37 centre (37.7, 2.9) radius 2.5
  circle A38 centre (2.9, 14.5) radius 2.5
  circle A39 centre (136.3, 2.9) radius 2.5
  circle A40 centre (107.3, 14.5) radius 2.5
  circle A41 centre (95.7, 26.1) radius 2.5
  circle A42 centre (136.3, 8.7) radius 2.5
  arc A43 (150, 2.9) -> (152.9, 0) centre (152.9, 2.9) ccw
  circle A44 centre (26.1, 31.9) radius 2.5
  circle A45 centre (14.5, 37.7) radius 2.5
  circle A46 centre (20.3, 2.9) radius 2.5
  circle A47 centre (113.1, 2.9) radius 2.5
  circle A48 centre (31.9, 2.9) radius 2.5
  circle A49 centre (26.1, 8.7) radius 2.5
  circle A50 centre (142.1, 14.5) radius 2.5
  circle A51 centre (14.5, 14.5) radius 2.5
  circle A52 centre (31.9, 20.3) radius 2.5
  circle A53 centre (113.1, 43.5) radius 2.5
  circle A54 centre (60.9, 20.3) radius 2.5
  circle A55 centre (43.5, 31.9) radius 2.5
  circle A56 centre (26.1, 2.9) radius 2.5
  arc A57 (167.5612, 0) -> (170, 2.4388) centre (167.5612, 2.4388) ccw
  circle A58 centre (55.1, 37.7) radius 2.5
  circle A59 centre (124.7, 2.9) radius 2.5
  circle A60 centre (136.3, 26.1) radius 2.5
  circle A61 centre (49.3, 14.5) radius 2.5
  circle A62 centre (136.3, 31.9) radius 2.5
  circle A63 centre (89.9, 26.1) radius 2.5
  circle A64 centre (130.5, 43.5) radius 2.5
  circle A65 centre (72.5, 20.3) radius 2.5
  circle A66 centre (78.3, 26.1) radius 2.5
  circle A67 centre (113.1, 26.1) radius 2.5
  circle A68 centre (155, 40) radius 2.5
  circle A69 centre (101.5, 8.7) radius 2.5
  circle A70 centre (78.3, 20.3) radius 2.5
  circle A71 centre (43.5, 37.7) radius 2.5
  circle A72 centre (72.5, 2.9) radius 2.5
  circle A73 centre (8.7, 43.5) radius 2.5
  circle A74 centre (14.5, 43.5) radius 2.5
  circle A75 centre (49.3, 43.5) radius 2.5
  circle A76 centre (2.9, 26.1) radius 2.5
  line L1 (170, 2.4388) -> (170, 43.0388)
  circle A77 centre (95.7, 8.7) radius 2.5
  circle A78 centre (107.3, 26.1) radius 2.5
  arc A79 (2.9, 49.3) -> (-2.9, 43.5) centre (2.9, 43.5) ccw
  circle A80 centre (124.7, 37.7) radius 2.5
  circle A81 centre (20.3, 26.1) radius 2.5
  arc A82 (170, 43.0388) -> (166.6388, 46.4) centre (166.6388, 43.0388) ccw
  circle A83 centre (118.9, 37.7) radius 2.5
  circle A84 centre (60.9, 43.5) radius 2.5
  circle A85 centre (20.3, 37.7) radius 2.5
  line L2 (0, 43.5) -> (0, 2.9)
  arc A86 (175, 43.5) -> (169.2, 49.3) centre (169.2, 43.5) ccw
  circle A87 centre (101.5, 20.3) radius 2.5
  circle A88 centre (66.7, 26.1) radius 2.5
  circle A89 centre (101.5, 14.5) radius 2.5
  circle A90 centre (101.5, 31.9) radius 2.5
  circle A91 centre (136.3, 37.7) radius 2.5
  circle A92 centre (155, 40) radius 2.5
  circle A93 centre (163.5, 30) radius 2.5
  circle A94 centre (37.7, 26.1) radius 2.5
  circle A95 centre (60.9, 37.7) radius 2.5
  circle A96 centre (118.9, 43.5) radius 2.5
  circle A97 centre (37.7, 37.7) radius 2.5
  circle A98 centre (60.9, 8.7) radius 2.5
  circle A99 centre (101.5, 37.7) radius 2.5
  circle A100 centre (60.9, 2.9) radius 2.5
  circle A101 centre (72.5, 26.1) radius 2.5
  arc A102 (2.9, 46.4) -> (0, 43.5) centre (2.9, 43.5) ccw
  circle A103 centre (72.5, 8.7) radius 2.5
  circle A104 centre (95.7, 37.7) radius 2.5
  circle A105 centre (89.9, 20.3) radius 2.5
  circle A106 centre (113.1, 20.3) radius 2.5
  circle A107 centre (66.7, 2.9) radius 2.5
  circle A108 centre (8.7, 31.9) radius 2.5
  circle A109 centre (60.9, 31.9) radius 2.5
  circle A110 centre (72.5, 14.5) radius 2.5
  line L3 (175, 2.9) -> (175, 43.5)
  circle A111 centre (155, 30) radius 2.5
  circle A112 centre (78.3, 43.5) radius 2.5
  circle A113 centre (43.5, 2.9) radius 2.5
  circle A114 centre (113.1, 37.7) radius 2.5
  circle A115 centre (43.5, 43.5) radius 2.5
  circle A116 centre (124.7, 26.1) radius 2.5
  circle A117 centre (66.7, 14.5) radius 2.5
  circle A118 centre (89.9, 8.7) radius 2.5
  circle A119 centre (124.7, 8.7) radius 2.5
  circle A120 centre (142.1, 31.9) radius 2.5
  circle A121 centre (142.1, 37.7) radius 2.5
  circle A122 centre (84.1, 37.7) radius 2.5
  circle A123 centre (2.9, 43.5) radius 2.5
  circle A124 centre (107.3, 2.9) radius 2.5
  circle A125 centre (37.7, 43.5) radius 2.5
  circle A126 centre (72.5, 43.5) radius 2.5
  circle A127 centre (78.3, 14.5) radius 2.5
  circle A128 centre (163.5, 20) radius 2.5
  circle A129 centre (55.1, 8.7) radius 2.5
  circle A130 centre (55.1, 31.9) radius 2.5
  circle A131 centre (84.1, 31.9) radius 2.5
  circle A132 centre (31.9, 43.5) radius 2.5
  circle A133 centre (49.3, 20.3) radius 2.5
  circle A134 centre (130.5, 26.1) radius 2.5
  circle A135 centre (95.7, 31.9) radius 2.5
  circle A136 centre (101.5, 2.9) radius 2.5
  circle A137 centre (55.1, 2.9) radius 2.5
  circle A138 centre (89.9, 37.7) radius 2.5
  circle A139 centre (107.3, 20.3) radius 2.5
  circle A140 centre (72.5, 37.7) radius 2.5
  circle A141 centre (14.5, 31.9) radius 2.5
  circle A142 centre (31.9, 37.7) radius 2.5
  circle A143 centre (113.1, 14.5) radius 2.5
  circle A144 centre (155, 20) radius 2.5
  circle A145 centre (14.5, 26.1) radius 2.5
  circle A146 centre (14.5, 8.7) radius 2.5
  circle A147 centre (49.3, 26.1) radius 2.5
  circle A148 centre (31.9, 8.7) radius 2.5
  arc A149 (169.2, -2.9) -> (175, 2.9) centre (169.2, 2.9) ccw
  circle A150 centre (55.1, 14.5) radius 2.5
  circle A151 centre (8.7, 26.1) radius 2.5
  circle A152 centre (2.9, 8.7) radius 2.5
  circle A153 centre (118.9, 20.3) radius 2.5
  circle A154 centre (43.5, 20.3) radius 2.5
  circle A155 centre (26.1, 26.1) radius 2.5
  circle A156 centre (66.7, 20.3) radius 2.5
  circle A157 centre (78.3, 8.7) radius 2.5
  circle A158 centre (107.3, 8.7) radius 2.5
  circle A159 centre (84.1, 43.5) radius 2.5
  circle A160 centre (14.5, 20.3) radius 2.5
  circle A161 centre (107.3, 31.9) radius 2.5
  circle A162 centre (78.3, 37.7) radius 2.5
  circle A163 centre (37.7, 8.7) radius 2.5
  circle A164 centre (130.5, 14.5) radius 2.5
  circle A165 centre (84.1, 20.3) radius 2.5
  circle A166 centre (136.3, 14.5) radius 2.5
  circle A167 centre (107.3, 43.5) radius 2.5
  circle A168 centre (78.3, 31.9) radius 2.5
  circle A169 centre (20.3, 8.7) radius 2.5
  circle A170 centre (49.3, 31.9) radius 2.5
  circle A171 centre (49.3, 8.7) radius 2.5
  circle A172 centre (66.7, 8.7) radius 2.5
  line L4 (145, 2.9) -> (145, 43.5)
  circle A173 centre (101.5, 26.1) radius 2.5
  line L5 (150, 43.5) -> (150, 2.9)
  circle A174 centre (130.5, 37.7) radius 2.5
  circle A175 centre (60.9, 26.1) radius 2.5
  circle A176 centre (118.9, 31.9) radius 2.5
  circle A177 centre (20.3, 43.5) radius 2.5
  circle A178 centre (55.1, 26.1) radius 2.5
  arc A179 (152.9, 46.4) -> (150, 43.5) centre (152.9, 43.5) ccw
  circle A180 centre (66.7, 43.5) radius 2.5
  circle A181 centre (89.9, 31.9) radius 2.5
  circle A182 centre (118.9, 8.7) radius 2.5
  arc A183 (145, 43.5) -> (142.1, 46.4) centre (142.1, 43.5) ccw
  circle A184 centre (142.1, 26.1) radius 2.5
  circle A185 centre (26.1, 37.7) radius 2.5
  circle A186 centre (49.3, 37.7) radius 2.5
  circle A187 centre (118.9, 26.1) radius 2.5
  circle A188 centre (84.1, 14.5) radius 2.5
  circle A189 centre (142.1, 43.5) radius 2.5
  circle A190 centre (124.7, 43.5) radius 2.5
  circle A191 centre (2.9, 31.9) radius 2.5
  circle A192 centre (8.7, 37.7) radius 2.5
  circle A193 centre (66.7, 31.9) radius 2.5
  circle A194 centre (136.3, 43.5) radius 2.5
  circle A195 centre (124.7, 14.5) radius 2.5
  circle A196 centre (118.9, 14.5) radius 2.5
  circle A197 centre (163.5, 40) radius 2.5
  circle A198 centre (84.1, 26.1) radius 2.5
  circle A199 centre (55.1, 43.5) radius 2.5
  circle A200 centre (43.5, 14.5) radius 2.5
  circle A201 centre (2.9, 37.7) radius 2.5
  circle A202 centre (72.5, 31.9) radius 2.5
  circle A203 centre (113.1, 31.9) radius 2.5
  circle A204 centre (20.3, 31.9) radius 2.5
  circle A205 centre (107.3, 37.7) radius 2.5
  circle A206 centre (37.7, 31.9) radius 2.5
  circle A207 centre (118.9, 2.9) radius 2.5
  circle A208 centre (113.1, 8.7) radius 2.5
  line L6 (166.6388, 46.4) -> (152.9, 46.4)
  circle A209 centre (43.5, 8.7) radius 2.5
  circle A210 centre (66.7, 37.7) radius 2.5
  circle A211 centre (89.9, 43.5) radius 2.5
  circle A212 centre (49.3, 2.9) radius 2.5
  circle A213 centre (26.1, 43.5) radius 2.5
  circle A214 centre (101.5, 43.5) radius 2.5
  circle A215 centre (155, 30) radius 2.5
  circle A216 centre (43.5, 26.1) radius 2.5
  circle A217 centre (55.1, 20.3) radius 2.5
  circle A218 centre (84.1, 2.9) radius 2.5
  circle A219 centre (130.5, 31.9) radius 2.5
  circle A220 centre (95.7, 14.5) radius 2.5
  circle A221 centre (31.9, 26.1) radius 2.5
  line L7 (2.9, 0) -> (142.1, 0)
  line L8 (142.1, 46.4) -> (2.9, 46.4)
  line L9 (169.2, 49.3) -> (2.9, 49.3)
  line L10 (2.9, -2.9) -> (169.2, -2.9)
  line L11 (-2.9, 43.5) -> (-2.9, 2.9)
  line L12 (177, 2.9) -> (177, 43.5)
  arc A222 (177, 43.5) -> (169.2, 51.3) centre (169.2, 43.5) ccw
  line L13 (169.2, 51.3) -> (2.9, 51.3)
  arc A223 (2.9, 51.3) -> (-4.9, 43.5) centre (2.9, 43.5) ccw
  line L14 (-4.9, 43.5) -> (-4.9, 2.9)
  arc A224 (-4.9, 2.9) -> (2.9, -4.9) centre (2.9, 2.9) ccw
  line L15 (2.9, -4.9) -> (169.2, -4.9)
  arc A225 (169.2, -4.9) -> (177, 2.9) centre (169.2, 2.9) ccw
  dimension "d23" = 2
  constraint horizontal L7
  constraint vertical L4
  constraint vertical L2
  constraint vertical L11
  constraint horizontal L10
  constraint horizontal L8
  constraint vertical L3
  constraint horizontal L9
  constraint tangent A79 L11
  constraint tangent A79 L9
  constraint tangent A29 L10
  constraint tangent A29 L11
  constraint tangent A149 L10
  constraint tangent L3 A149
  constraint tangent A86 L9
  constraint tangent A86 L3
  constraint tangent L2 A102
  constraint tangent A102 L8
  constraint tangent A11 L2
  constraint tangent A11 L7
  constraint tangent A10 L7
  constraint tangent A10 L4
  constraint tangent A183 L8
  constraint tangent L4 A183
  constraint horizontal L0
  constraint vertical L1
  constraint horizontal L6
  constraint tangent L0 A57
  constraint tangent A57 L1
  constraint tangent A82 L6
  constraint tangent L1 A82
  constraint vertical L5
  constraint tangent L5 A179
  constraint tangent A43 L5
  constraint coincident L0.start L7
extrude "Extruir3" add sketch "Boceto4" along normal blind 2 contours L12 A222 L13 A223 L14 A224 L15 A225 bodies 2
